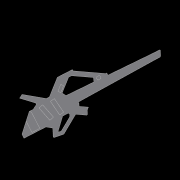
# Autodesk Inventor part: Hybrid
Saved by Autodesk Inventor 2020 (Build 240168000, 168)
## iProperties
Created: 2022-11-06
Part Number: Hybrid
Material: Generic
Document SubType Name: Modeling
Designer: Val
Density: 1 g/cm^3
Appearance: Default
Author: Val
Autodesk Inventor part; units mm, degrees
ref_plane "YZ Plane" through (0, 0, 0) normal (1, 0, 0) x (0, 1, 0)
ref_plane "XZ Plane" through (0, 0, 0) normal (0, 1, 0) x (-1, 0, 0)
ref_plane "XY Plane" through (0, 0, 0) normal (0, 0, 1) x (1, 0, 0)
sketch "Reference" plane through (0, 0, 0) normal (0, 0, 1) x (1, 0, 0)
  line L0 (-265.1838, 66.2948) -> (610.5672, 45.41)
  line L1 (-253.4935, -33.7986) -> (584.2, -11.1347)
  line L2 (610.5672, 45.41) -> (584.2, -11.1347)
  line L3 (-265.1838, 66.2948) -> (-253.4935, -33.7986) construction
  line L4 (-330.2, 87.8141) -> (-370.5371, 82.8613)
  line L5 (-370.5371, 82.8613) -> (-353.5119, -55.7974)
  line L6 (-353.5119, -55.7974) -> (-313.1749, -50.8446)
  line L7 (-313.1749, -50.8446) -> (-330.2, 87.8141)
  line L8 (0, -84.2353) -> (0, 115.8314) construction
  line L9 (-442.9271, 87.2481) -> (-482.3599, 77.4164)
  line L10 (-482.3599, 77.4164) -> (-448.5634, -58.1339)
  line L11 (-448.5634, -58.1339) -> (-409.1306, -48.3022)
  line L12 (-409.1306, -48.3022) -> (-442.9271, 87.2481)
  line L13 (-612.775, 70.027) -> (-533.4, 70.027)
  line L14 (-533.4, 70.027) -> (-533.4, 52.247) construction
  line L15 (-533.4, 52.247) -> (-612.775, 52.247)
  line L16 (-612.775, 52.247) -> (-612.775, 70.027)
  circle A0 centre (-533.4, 61.137) radius 8.89
  line L17 (-612.775, 70.027) -> (-630.555, 70.027)
  line L18 (-630.555, 70.027) -> (-630.555, 52.247)
  line L19 (-630.555, 52.247) -> (-612.775, 52.247)
  line L20 (-612.775, 52.247) -> (-612.775, 70.027)
  line L21 (-533.4, 61.137) -> (-477.9163, -57.8481) construction
  line L22 (-635, 228.6) -> (0, 228.6) construction
  line L23 (0, 228.6) -> (0, -209.55) construction
  line L24 (0, -209.55) -> (-635, -209.55) construction
  line L25 (-635, -209.55) -> (-635, 228.6) construction
  line L26 (610.5672, 45.41) -> (643.2113, 45.41)
  line L27 (643.2113, 45.41) -> (643.2113, 38.7509)
  line L28 (643.2113, 38.7509) -> (602.1746, -11.1347)
  line L29 (602.1746, -11.1347) -> (584.2, -11.1347)
  line L30 (-533.4, 61.137) -> (623.244, 37.4869) construction
  line L31 (-521.6688, 35.9793) -> (616.4636, 32.1556) construction
  line L32 (-511.3831, 13.9215) -> (611.3127, 20.8416) construction
  line L33 (-499.7799, -10.9615) -> (605.289, 10.3914) construction
  line L34 (-489.2369, -33.5711) -> (600.1336, -0.0544) construction
  circle A1 centre (-521.6688, 35.9793) radius 8.89
  circle A2 centre (-511.3831, 13.9215) radius 8.89
  circle A3 centre (-499.7799, -10.9615) radius 8.89
  circle A4 centre (-489.2369, -33.5711) radius 8.89
  circle A5 centre (-337.8933, -92.7495) radius 12.7
  line L35 (0, 203.2) -> (-635, 203.2) construction
  line L36 (-635, 203.2) -> (-635, -158.75) construction
  line L37 (-635, -158.75) -> (0, -158.75) construction
  line L38 (0, -158.75) -> (0, 203.2) construction
  line L39 (-635, -127) -> (0, -127) construction
  line L40 (0, -127) -> (0, 152.4) construction
  line L41 (0, 152.4) -> (-635, 152.4) construction
  line L42 (-635, 152.4) -> (-635, -127) construction
  line L43 (-521.6688, 44.8693) -> (-601.0438, 44.8693)
  line L44 (-601.0438, 44.8693) -> (-601.0438, 27.0893)
  line L45 (-601.0438, 27.0893) -> (-521.6688, 27.0893)
  line L46 (-521.6688, 27.0893) -> (-521.6688, 44.8693) construction
  line L47 (-601.0438, 44.8693) -> (-618.8238, 44.8693)
  line L48 (-618.8238, 44.8693) -> (-618.8238, 27.0893)
  line L49 (-618.8238, 27.0893) -> (-601.0438, 27.0893)
  line L50 (-601.0438, 27.0893) -> (-601.0438, 44.8693)
  line L51 (-511.3831, 22.8115) -> (-590.7581, 22.8115)
  line L52 (-590.7581, 22.8115) -> (-590.7581, 5.0315)
  line L53 (-590.7581, 5.0315) -> (-511.3831, 5.0315)
  line L54 (-511.3831, 5.0315) -> (-511.3831, 22.8115) construction
  line L55 (-590.7581, 22.8115) -> (-608.5381, 22.8115)
  line L56 (-608.5381, 22.8115) -> (-608.5381, 5.0315)
  line L57 (-608.5381, 5.0315) -> (-590.7581, 5.0315)
  line L58 (-590.7581, 5.0315) -> (-590.7581, 22.8115)
  line L59 (-499.7799, -2.0715) -> (-579.1549, -2.0715)
  line L60 (-579.1549, -2.0715) -> (-579.1549, -19.8515)
  line L61 (-579.1549, -19.8515) -> (-499.7799, -19.8515)
  line L62 (-499.7799, -19.8515) -> (-499.7799, -2.0715) construction
  line L63 (-579.1549, -2.0715) -> (-596.9349, -2.0715)
  line L64 (-596.9349, -2.0715) -> (-596.9349, -19.8515)
  line L65 (-596.9349, -19.8515) -> (-579.1549, -19.8515)
  line L66 (-579.1549, -19.8515) -> (-579.1549, -2.0715)
  line L67 (-489.2369, -24.6811) -> (-568.6119, -24.6811)
  line L68 (-568.6119, -24.6811) -> (-568.6119, -42.4611)
  line L69 (-568.6119, -42.4611) -> (-489.2369, -42.4611)
  line L70 (-489.2369, -42.4611) -> (-489.2369, -24.6811)
  line L71 (-568.6119, -24.6811) -> (-586.3919, -24.6811)
  line L72 (-586.3919, -24.6811) -> (-586.3919, -42.4611)
  line L73 (-586.3919, -42.4611) -> (-568.6119, -42.4611)
  line L74 (-568.6119, -42.4611) -> (-568.6119, -24.6811)
  point P0 (0, 0)
  dimension "d148" = 25.4
  dimension "d149" = 17.78
  dimension "d150" = 140.559
  dimension "d151" = 25
  dimension "d152" = 91.366
  dimension "d153" = 91.55
  dimension "d154" = 91.762
  dimension "d155" = 91.107
  dimension "d156" = 90.353
  dimension "d157" = 89.808
  dimension "d158" = 88.829
  dimension "d159" = 6.662
  dimension "d160" = 7
  dimension "d161" = 14
  dimension "d162" = 25
  dimension "d163" = 643.2113
  dimension "d164" = 1132.4481
  dimension "d165" = 1142.9912
  dimension "d166" = 1154.5943
  dimension "d167" = 1164.88
  dimension "d168" = 1176.6113
  dimension "d169" = 1211.8231
  dimension "d170" = 1229.6031
  dimension "d171" = 1278.2113
  dimension "d172" = 56.5447
  dimension "d173" = 183.19
  dimension "d174" = 254.96
  dimension "d175" = 157.79
  dimension "d176" = 204.16
  dimension "d177" = 47.4815
  dimension "d178" = 106.99
  dimension "d179" = 172.41
  dimension "d180" = 40.64
  dimension "d181" = 139.7
  dimension "d182" = 4.2304
  dimension "d183" = 29.5856
  dimension "d184" = 899.8393
  dimension "d185" = 960.9878
  dimension "d186" = 21.017
  dimension "d187" = 1043.7538
  dimension "d188" = 163.656
  dimension "d189" = 19.9673
  dimension "d190" = 26.7477
  dimension "d191" = 31.8986
  dimension "d192" = 37.9222
  dimension "d193" = 43.0776
  dimension "d194" = 70.4214
  dimension "d195" = 643.2113
  dimension "d196" = 45.41
  dimension "d197" = 129.6453
  dimension "d198" = 981.1046
  dimension "d199" = 138.1595
  dimension "d200" = 1121.1276
  constraints: 150 end point, 31 parallel, 18 perpendicular, 14 horizontal, 10 equal length, 8 collinear, 8 point on circle, 6 centre point, 5 point on line, 5 tangent, 4 coincident, 4 equal radius, 1 midpoint
  measures "d148" diameter of A5
  measures "d149" diameter of A4
  measures "d150" angle of L27 L28
  measures "d151" angle of L27 L2
  measures "d152" angle of L27 L0
  measures "d153" angle of L27 L1
  measures "d154" angle of L34 L27
  measures "d155" angle of L33 L27
  measures "d156" angle of L32 L27
  measures "d157" angle of L31 L27
  measures "d158" angle of L30 L27
  measures "d159" angle of L27 L3
  measures "d160" angle of L27 L7
  measures "d161" angle of L27 L12
  measures "d162" angle of L27 L21
  measures "d163" distance between parallel lines of L27 L23
  measures "d164" distance between parallel lines of L27 L70
  measures "d165" distance between parallel lines of L27 L62
  measures "d166" distance between parallel lines of L27 L54
  measures "d167" distance between parallel lines of L27 L46
  measures "d168" distance between parallel lines of L27 L14
  measures "d169" distance between parallel lines of L27 L68
  measures "d170" distance between parallel lines of L27 L72
  measures "d171" distance between parallel lines of L27 L25
  measures "d172" distance between parallel lines of L26 L29
  measures "d173" distance between parallel lines of L26 L22
  measures "d174" distance between parallel lines of L26 L24
  measures "d175" distance between parallel lines of L26 L35
  measures "d176" distance between parallel lines of L26 L37
  measures "d177" distance between parallel lines of L26 L59
  measures "d178" distance between parallel lines of L26 L41
  measures "d179" distance between parallel lines of L26 L39
  measures "d180" distance between parallel lines of L7 L5
  measures "d181" distance between parallel lines of L6 L4
  measures "d182" distance from line of L26.end L28
  measures "d183" distance from line of L26.end L2
  measures "d184" distance from line of L26.end L3
  measures "d185" distance from line of L26.end L7
  measures "d186" distance from line of L26.end L6
  measures "d187" distance from line of L26.end L12
  measures "d188" distance from line of L26.end L11
  measures "d189" distance from line of L30.end L27
  measures "d190" distance from line of L31.end L27
  measures "d191" distance from line of L32.end L27
  measures "d192" distance from line of L33.end L27
  measures "d193" distance from line of L34.end L27
  measures "d194" distance from line of L8.end L26
  measures "d195" distance from line of point (0, 0) L27
  measures "d196" distance from line of point (0, 0) L26
  measures "d197" distance from line of L8.start L26
  measures "d198" distance from line of A5.centre L27
  measures "d199" distance from line of A5.centre L26
  measures "d200" distance from line of L21.end L27
sketch "Body" plane through (0, 0, 0) normal (0, 0, 1) x (1, 0, 0)
  line L0 (-265.1838, 66.2948) -> (610.5672, 45.41)
  line L1 (-253.4935, -33.7986) -> (584.2, -11.1347)
  line L2 (-302.7546, -14.2759) -> (-288.4229, -34.7436)
  line L3 (-253.4935, -33.7986) -> (-288.4229, -34.7436)
  line L4 (-265.1838, 66.2948) -> (-302.7546, -14.2759)
  line L5 (-249.8117, 99.3456) -> (-231.3256, 65.4874)
  line L6 (-249.8117, 99.3456) -> (-139.6504, 193.8782)
  line L7 (-361.5717, 119.38) -> (-390.1467, 119.38)
  line L8 (-361.5717, 119.38) -> (-224.4383, 237.0582)
  line L9 (-224.4383, 237.0582) -> (-89.3317, 237.0582)
  line L10 (-139.6504, 193.8782) -> (-111.0754, 193.8782)
  line L11 (-111.0754, 193.8782) -> (46.8805, 95.1764)
  line L12 (-89.3317, 237.0582) -> (166.2104, 77.3778) construction
  line L13 (46.8805, 95.1764) -> (33.7735, 59.1653)
  line L14 (610.5672, 45.41) -> (584.2, -11.1347)
  line L15 (-139.6504, 193.8782) -> (-89.3317, 237.0582) construction
  line L16 (-390.1467, 119.38) -> (-557.5007, 245.4903)
  line L17 (-531.8838, 88.9) -> (-569.9838, 88.9)
  line L18 (-569.9838, 88.9) -> (-713.6679, -54.7841)
  line L19 (-713.6679, -54.7841) -> (-713.6679, -92.8841)
  line L20 (-456.7922, -128.5466) -> (-491.6793, -203.3623)
  line L21 (-491.6793, -203.3623) -> (-397.4756, -217.4411)
  line L22 (-397.4756, -217.4411) -> (-230.5373, -113.1265)
  line L23 (-556.0382, 74.9544) -> (-556.0382, -80.1841)
  line L24 (-556.0382, -80.1841) -> (-631.1179, -80.1841)
  line L25 (-631.1179, -80.1841) -> (-631.1179, 27.7659)
  line L26 (-631.1179, 27.7659) -> (-569.9838, 88.9)
  line L27 (-569.9838, 88.9) -> (-556.0382, 74.9544)
  line L28 (-487.8897, 114.3) -> (-531.8838, 88.9)
  line L29 (-713.6679, -92.8841) -> (-504.1179, -92.8841)
  line L30 (-504.1179, -92.8841) -> (-456.7922, -128.5466)
  line L31 (-556.0382, 74.9544) -> (-531.8838, 88.9) construction
  line L32 (-487.8897, 114.3) -> (-487.8897, 127)
  line L33 (-557.5007, 245.4903) -> (-590.4963, 226.4403)
  line L34 (-487.8897, 127) -> (-590.4963, 226.4403)
  line L35 (-163.0546, -31.3518) -> (-163.0546, -44.0518)
  line L36 (-163.0546, -44.0518) -> (-173.7891, -67.072)
  line L37 (-173.7891, -67.072) -> (-106.4752, -109.1343)
  line L38 (-230.5373, -113.1265) -> (-144.8632, -166.6617)
  line L39 (-125.751, -125.6754) -> (-144.8632, -166.6617)
  line L40 (-106.4752, -109.1343) -> (-125.751, -125.6754)
  line L41 (166.2104, 77.3778) -> (165.701, 56.0191)
  line L42 (610.5672, 45.41) -> (661.3672, 45.41)
  line L43 (584.2, -11.1347) -> (635, -11.1347)
  line L44 (661.3672, 45.41) -> (635, -11.1347)
  line L45 (-89.3317, 237.0582) -> (-80.8735, 237.0582)
  line L46 (-80.8735, 237.0582) -> (-80.8735, 224.3582)
  line L47 (-80.8735, 224.3582) -> (154.3443, 77.3778)
  line L48 (154.3443, 77.3778) -> (166.2104, 77.3778)
  line L49 (-284.4959, -109.4047) -> (-273.8634, -86.6032)
  line L50 (-273.8634, -86.6032) -> (-281.1479, -76.2)
  line L51 (-281.1479, -76.2) -> (-335.5425, -76.2)
  line L52 (-335.5425, -76.2) -> (-428.2379, -172.1889)
  line L53 (-428.2379, -172.1889) -> (-429.4881, -180.5542)
  line L54 (-429.4881, -180.5542) -> (-404.3671, -184.3086)
  line L55 (-404.3671, -184.3086) -> (-284.4959, -109.4047)
  line L56 (-988.6749, 0) -> (936.3742, 0) construction
  line L57 (0, -310.0274) -> (0, 338.0766) construction
  line L58 (-533.4, 61.137) -> (623.244, 37.4869) construction
  line L59 (-521.6688, 35.9793) -> (616.4636, 32.1556) construction
  line L60 (-511.3831, 13.9215) -> (611.3127, 20.8416) construction
  line L61 (-499.7799, -10.9615) -> (605.289, 10.3914) construction
  line L62 (-489.2369, -33.5711) -> (600.1336, -0.0544) construction
  line L63 (-442.9271, 87.2481) -> (-482.3599, 77.4164) projected
  line L64 (-482.3599, 77.4164) -> (-448.5634, -58.1339) projected
  line L65 (-409.1306, -48.3022) -> (-442.9271, 87.2481) projected
  line L66 (-448.5634, -58.1339) -> (-409.1306, -48.3022) projected
  line L67 (-330.2, 87.8141) -> (-370.5371, 82.8613) projected
  line L68 (-370.5371, 82.8613) -> (-353.5119, -55.7974) projected
  line L69 (-313.1749, -50.8446) -> (-330.2, 87.8141) projected
  line L70 (-353.5119, -55.7974) -> (-313.1749, -50.8446) projected
  circle A0 centre (-533.4, 61.137) radius 8.89 construction
  line L71 (-612.775, 70.027) -> (-533.4, 70.027) construction
  line L72 (-533.4, 52.247) -> (-612.775, 52.247) construction
  line L73 (-612.775, 52.247) -> (-612.775, 70.027) construction
  line L74 (-630.555, 70.027) -> (-630.555, 52.247) construction
  line L75 (-612.775, 70.027) -> (-630.555, 70.027) construction
  line L76 (-630.555, 52.247) -> (-612.775, 52.247) construction
  line L77 (-618.8238, 44.8693) -> (-618.8238, 27.0893) construction
  line L78 (-601.0438, 44.8693) -> (-618.8238, 44.8693) construction
  line L79 (-618.8238, 27.0893) -> (-601.0438, 27.0893) construction
  line L80 (-601.0438, 27.0893) -> (-601.0438, 44.8693) construction
  line L81 (-521.6688, 44.8693) -> (-601.0438, 44.8693) construction
  line L82 (-601.0438, 27.0893) -> (-521.6688, 27.0893) construction
  circle A1 centre (-521.6688, 35.9793) radius 8.89 construction
  circle A2 centre (-511.3831, 13.9215) radius 8.89 construction
  line L83 (-511.3831, 22.8115) -> (-590.7581, 22.8115) construction
  line L84 (-590.7581, 5.0315) -> (-511.3831, 5.0315) construction
  line L85 (-590.7581, 22.8115) -> (-590.7581, 5.0315) construction
  line L86 (-590.7581, 22.8115) -> (-608.5381, 22.8115) construction
  line L87 (-608.5381, 5.0315) -> (-590.7581, 5.0315) construction
  line L88 (-608.5381, 22.8115) -> (-608.5381, 5.0315) construction
  line L89 (-596.9349, -2.0715) -> (-596.9349, -19.8515) construction
  line L90 (-579.1549, -2.0715) -> (-596.9349, -2.0715) construction
  line L91 (-596.9349, -19.8515) -> (-579.1549, -19.8515) construction
  line L92 (-579.1549, -19.8515) -> (-579.1549, -2.0715) construction
  line L93 (-499.7799, -2.0715) -> (-579.1549, -2.0715) construction
  line L94 (-579.1549, -19.8515) -> (-499.7799, -19.8515) construction
  circle A3 centre (-499.7799, -10.9615) radius 8.89 construction
  circle A4 centre (-489.2369, -33.5711) radius 8.89 construction
  line L95 (-489.2369, -24.6811) -> (-568.6119, -24.6811) construction
  line L96 (-568.6119, -42.4611) -> (-489.2369, -42.4611) construction
  line L97 (-568.6119, -24.6811) -> (-568.6119, -42.4611) construction
  line L98 (-568.6119, -24.6811) -> (-586.3919, -24.6811) construction
  line L99 (-586.3919, -42.4611) -> (-568.6119, -42.4611) construction
  line L100 (-586.3919, -24.6811) -> (-586.3919, -42.4611) construction
  point P0 (0, 0)
  dimension "d51" = 88.9
  dimension "d54" = 33.8582
  dimension "d55" = 120
  dimension "d56" = 102
  dimension "d58" = 33.8582
  dimension "d60" = 43.18
  dimension "d61" = 148
  dimension "d62" = 28.575
  dimension "d63" = 186.2582
  dimension "d64" = 120.65
  dimension "d65" = 102
  dimension "d66" = 28.575
  dimension "d67" = 111.76
  dimension "d68" = 143
  dimension "d70" = 209.55
  dimension "d73" = 50.8
  dimension "d75" = 38.1
  dimension "d78" = 38.1
  dimension "d80" = 304.8
  dimension "d81" = 209.55
  dimension "d83" = 59.2582
  dimension "d85" = 82.55
  dimension "d88" = 95.25
  dimension "d89" = 196.85
  dimension "d93" = 120
  dimension "d94" = 82.55
  dimension "d95" = 12.7
  dimension "d96" = 38.1
  dimension "d97" = 12.7
  dimension "d98" = 139.7
  dimension "d99" = 12.7
  dimension "d100" = 25.4
  dimension "d101" = 79.375
  dimension "d102" = 25.4
  dimension "d104" = 50.8
  dimension "d105" = 8.4582
  dimension "d106" = 12.7
  dimension "d113" = 31.75
  dimension "d114" = 31.75
  dimension "d115" = 50.8
  dimension "d117" = 12.7
  dimension "d118" = 8.4582
  dimension "d119" = 14
  dimension "d120" = 25.4
  dimension "d127" = 44.102
  dimension "d128" = 40.634
  dimension "d129" = 45
  dimension "d130" = 65
  dimension "d131" = 46
  dimension "d132" = 54.5
  dimension "d134" = 1.55
  dimension "d135" = 115
  dimension "d136" = 56.5447
  dimension "d137" = 265.1838
  dimension "d138" = 66.2948
  dimension "d139" = 69.1284
  dimension "d140" = 134
  dimension "d141" = 50.4761
  dimension "d142" = 41.4564
  dimension "d143" = 135.1066
  dimension "d145" = 38.3222
  dimension "d146" = 113
  dimension "d147" = 37
  constraints: 112 end point, 20 parallel, 6 horizontal, 5 collinear, 4 perpendicular, 4 point on line, 3 vertical
  measures "d51" distance of L0.start L2.start
  measures "d54" horizontal distance of L0.start L5.end
  measures "d55" angle of L0 L5
  measures "d56" angle of L6 L5
  measures "d58" vertical distance of L5.end L5.start
  measures "d60" distance between parallel lines of L9 L10
  measures "d61" angle of L11 L10
  measures "d62" distance of L10.end L6.end
  measures "d63" distance of L10.end L11.end
  measures "d64" distance of L11.end L12.end
  measures "d65" angle of L11 L13
  measures "d66" distance of L7.start L7.end
  measures "d67" horizontal distance of L5.start L7.start
  measures "d68" angle of L16 L7
  measures "d70" distance of L7.end L16.end
  measures "d73" distance of L28.start L17.start
  measures "d75" distance of L17.start L17.end
  measures "d78" distance of L18.end L19.end
  measures "d80" horizontal distance of L0.start L17.end
  measures "d81" distance of L19.end L29.end
  measures "d83" distance of L29.end L20.start
  measures "d85" distance of L20.start L20.end
  measures "d88" distance of L20.end L21.end
  measures "d89" distance of L21.end L22.end
  measures "d93" angle of L4 L2
  measures "d94" distance between parallel lines of L19 L25
  measures "d95" distance between parallel lines of L29 L24
  measures "d96" distance of L16.end L33.end
  measures "d97" distance of L28.start L32.end
  measures "d98" horizontal distance of L2.start L35.start
  measures "d99" distance of L35.start L35.end
  measures "d100" distance of L35.end L36.end
  measures "d101" distance of L36.end L37.end
  measures "d102" distance of L37.end L39.start
  measures "d104" distance of L0.end L42.end
  measures "d105" distance of L9.end L45.end
  measures "d106" distance of L45.end L46.end
  measures "d113" distance between parallel lines of L22 L55
  measures "d114" distance between parallel lines of L21 L54
  measures "d115" distance of L22.end L49.end
  measures "d117" distance of L49.end L50.end
  measures "d118" distance of L52.end L53.end
  measures "d119" angle of L55 L52
  measures "d120" distance of L53.end L54.end
  measures "d127" angle of L56 L34
  measures "d128" angle of L56 L8
  measures "d129" angle of L18 L56
  measures "d130" angle of L56 L4
  measures "d131" angle of L52 L56
  measures "d132" angle of L52 L54
  measures "d134" angle of L1 L56
  measures "d135" angle of L56 L14
  measures "d136" distance between parallel lines of L43 L42
  measures "d137" distance from line of L57 L0.start
  measures "d138" vertical distance of point (0, 0) L0.start
  measures "d139" distance between parallel lines of L38 L37
  measures "d140" angle of L51 L52
  measures "d141" distance from line of L22.end L49
  measures "d142" distance from line of L2.end L51
  measures "d143" distance of L8.end L9.end
  measures "d145" distance of L11.end L13.end
  measures "d146" angle of L16 L33
  measures "d147" angle of L56 L16
extrude "BodyFeature" add sketch "Body" along normal blind 38.1 contours L4 L2 L3 L1 L35 L36 L37 L40 L39 L38 L22 L21 L20 L30 L29 L19 L18 L25 L24 L23 L27 L17 L28 L32 L34 L33 L16 L7 L8 L9 L45 L46 L47 L48 L41 L0 L13 L11 L10 L6 L5 | L0 L14 L1 L3 L2 L4 | L42 L44 L43 L14 | L27 L23 L24 L25 L18 | L65 L66 L64 L63 | L69 L70 L68 L67
sketch "TunersIndentation" plane through (0, 0, 38.1) normal (0, 0, 1) x (1, 0, 0)
  line L0 (-569.9838, 88.9) -> (-556.0382, 74.9544) projected
  line L1 (-556.0382, 74.9544) -> (-556.0382, -80.1841) projected
  line L2 (-556.0382, -80.1841) -> (-631.1179, -80.1841) projected
  line L3 (-631.1179, -80.1841) -> (-631.1179, 27.7659) projected
  line L4 (-631.1179, 27.7659) -> (-569.9838, 88.9) projected
  point P0 (0, 0)
extrude "TunersIndentationFeature" cut sketch "TunersIndentation" against normal blind 8
chamfer "TunersChamferFeature" distance 3.175 angle 45 2 edges at (-556.0382, -80.1841, 34.1) (-631.1179, -80.1841, 34.1)
sketch "Detail" plane through (0, 0, 38.1) normal (0, 0, 1) x (1, 0, 0)
  line L0 (67.6317, 87.5399) -> (102.8869, 87.5399)
  line L1 (102.8869, 87.5399) -> (102.8869, 57.5171)
  line L2 (102.8869, 57.5171) -> (67.6317, 57.5171)
  line L3 (67.6317, 57.5171) -> (67.6317, 87.5399)
  line L4 (-224.4383, 237.0582) -> (-361.5717, 119.38) construction
  line L5 (-275.136, 128.8567) -> (-226.9467, 170.2094)
  line L6 (-226.9467, 170.2094) -> (-209.8929, 150.3361)
  line L7 (-209.8929, 150.3361) -> (-258.0822, 108.9835)
  line L8 (-258.0822, 108.9835) -> (-275.136, 128.8567)
  line L9 (-275.136, 128.8567) -> (-209.8929, 150.3361) construction
  line L10 (-226.9467, 170.2094) -> (-258.0822, 108.9835) construction
  line L11 (-132.8355, 39.6875) -> (26.6842, 39.6875) construction
  line L12 (26.6842, 39.6875) -> (26.6842, 3.8778) construction
  line L13 (26.6842, 3.8778) -> (-132.8355, 3.8778) construction
  line L14 (-132.8355, 3.8778) -> (-132.8355, 39.6875) construction
  line L15 (-249.8117, 99.3456) -> (-139.6504, 193.8782) construction
  line L16 (-249.8117, 99.3456) -> (-307.1092, 166.1159) construction
  line L17 (-240.0112, 124.4907) -> (-238.9691, 123.2763)
  line L18 (-238.9691, 123.2763) -> (-226.9218, 133.6145)
  line L19 (-226.9218, 133.6145) -> (-227.9639, 134.8289)
  line L20 (-232.9455, 128.4454) -> (-242.5145, 139.5964) construction
  circle A0 centre (69.2192, 85.9524) radius 1.5875
  circle A1 centre (101.2994, 85.9524) radius 1.5875
  circle A2 centre (101.2994, 59.1046) radius 1.5875
  circle A3 centre (69.2192, 59.1046) radius 1.5875
  line L21 (46.8805, 95.1764) -> (33.7735, 59.1653) construction
  line L22 (33.7735, 59.1653) -> (165.701, 56.0191) construction
  line L23 (46.8805, 95.1764) -> (166.1637, 75.4202) construction
  line L24 (165.701, 56.0191) -> (166.2104, 77.3778) construction
  line L25 (33.7735, 59.1653) -> (26.6842, 39.6875) construction
  point P0 (154.3443, 77.3778)
  point P1 (69.2192, 57.5171)
  point P2 (101.2994, 57.5171)
  point P3 (102.8869, 59.1046)
  point P4 (102.8869, 85.9524)
  point P5 (101.2994, 87.5399)
  point P6 (69.2192, 87.5399)
  point P7 (67.6317, 85.9524)
  point P8 (67.6317, 59.1046)
  dimension "d209" = 63.5
  dimension "d210" = 26.1874
  dimension "d211" = 12.7
  dimension "d212" = 15.875
  dimension "d213" = 1.6002
  dimension "d220" = 35.2552
  dimension "d221" = 30.0228
  dimension "d223" = 3.175
  dimension "d224" = 33.8582
  dimension "d225" = 0
  dimension "d229" = 19.4778
  constraints: 44 end point, 8 perpendicular, 8 tangent, 6 parallel, 5 point on line, 4 centre point, 3 equal radius, 3 midpoint, 2 collinear, 2 horizontal, 1 coincident
  measures "d209" distance of L5.start L5.end
  measures "d210" distance of L7.end L5.start
  measures "d211" distance between parallel lines of L15 L7
  measures "d212" distance of L17.end L18.end
  measures "d213" distance of L18.end L19.end
  measures "d220" distance of L0.start L0.end
  measures "d221" distance of L2.end L0.start
  measures "d223" diameter of A0
  measures "d224" horizontal distance of L21.end L2.end
  measures "d225" distance from line of L22 L1.end
  measures "d229" distance from line of L11 L21.end
extrude "OscCutFeature" cut sketch "Detail" against normal blind 8 contours L5 L6 L7 L8 | L7 L19 L18 L17
fillet "OscSmallFilletsFeature" radius 0.254 6 edges at (-226.9467, 170.2094, 34.1) (-275.136, 128.8567, 34.1) (-209.8929, 150.3361, 34.1) (-258.0822, 108.9835, 34.1) (-240.0112, 124.4907, 34.1) (-227.9639, 134.8289, 34.1)
fillet "OscLargeFilletsFeature" radius 1.524 2 edges at (-238.9691, 123.2763, 34.1) (-226.9218, 133.6145, 34.1)
extrude "LogoCutFeature" cut sketch "Detail" against normal blind 8 contours L0 A1 L1 A2 L2 A3 L3 A0
fillet "LogoCutFilletsFeature" radius 2.54 8 edges at (102.8869, 85.9524, 34.1) (101.2994, 87.5399, 34.1) (101.2994, 57.5171, 34.1) (102.8869, 59.1046, 34.1) (69.2192, 57.5171, 34.1) (67.6317, 59.1046, 34.1) (67.6317, 85.9524, 34.1) (69.2192, 87.5399, 34.1)
chamfer "BottomChamfers" distance 6.35 angle 45 2 edges at (-144.8632, -166.6617, 19.05) (-491.6793, -203.3623, 19.05)
chamfer "NeckChamfer" distance 6.35 angle 45 2 edges at (661.3672, 45.41, 19.05) (635, -11.1347, 19.05)
sketch "Pickups" plane through (0, 0, 38.1) normal (0, 0, 1) x (1, 0, 0)
  line L0 (-442.9271, 87.2481) -> (-482.3599, 77.4164) projected
  line L1 (-482.3599, 77.4164) -> (-448.5634, -58.1339) projected
  line L2 (-409.1306, -48.3022) -> (-442.9271, 87.2481) projected
  line L3 (-448.5634, -58.1339) -> (-409.1306, -48.3022) projected
  line L4 (-370.5371, 82.8613) -> (-353.5119, -55.7974) projected
  line L5 (-330.2, 87.8141) -> (-370.5371, 82.8613) projected
  line L6 (-353.5119, -55.7974) -> (-313.1749, -50.8446) projected
  line L7 (-313.1749, -50.8446) -> (-330.2, 87.8141) projected
  point P0 (0, 0)
extrude "PickupsFeature" add sketch "Pickups" along normal blind 6
fillet "PickupFilletsFeature" radius 3.175 8 edges at (-448.5634, -58.1339, 41.1) (-409.1306, -48.3022, 41.1) (-482.3599, 77.4164, 41.1) (-442.9271, 87.2481, 41.1) (-370.5371, 82.8613, 41.1) (-330.2, 87.8141, 41.1) (-353.5119, -55.7974, 41.1) (-313.1749, -50.8446, 41.1)
body "Solid1"
